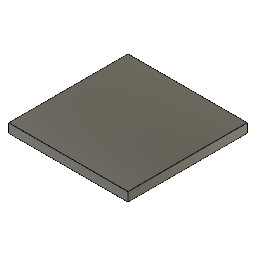
stepper_nema17 v0 (Autodesk Fusion 360 design; units mm, degrees)
Autodesk Fusion 360 part; units mm, degrees
sketch "Sketch1" plane through (0, 0, 0) normal (0, 0, 1) x (1, 0, 0)
  line L0 (21, -21) -> (-21, -21)
  line L1 (-21, -21) -> (-21, 21)
  line L2 (-21, 21) -> (21, 21)
  line L3 (21, 21) -> (21, -21)
  line L4 (21, -21) -> (-21, 21) construction
  line L5 (-21, -21) -> (21, 21) construction
  circle A0 centre (16, -16) radius 1.5
  line L6 (0, 0) -> (21, 0)
  line L7 (0, 0) -> (0, -21)
  line L8 (0, 0) -> (0, 21)
  line L9 (0, 0) -> (-21, 0)
  circle A1 centre (16, 16) radius 1.5
  circle A2 centre (-16, -16) radius 1.5
  circle A3 centre (-16, 16) radius 1.5
  dimension "d1" = 42
  dimension "d2" = 42
  dimension "d3" = 3
  dimension "d4" = 5
  dimension "d5" = 5
  constraint horizontal L0
  constraint perpendicular L0 L1
  constraint parallel L0 L2
  constraint parallel L1 L3
  constraint coincident L4 L6.start
  constraint coincident L5 L6.start
  constraint coincident L6.start L7.start
  constraint midpoint L3 L6.end
  constraint midpoint L0 L7.end
  constraint midpoint L2 L8.end
  constraint midpoint L1 L9.end
  constraint symmetric A0 L6 A1
  constraint symmetric A0 L7 A2
  constraint symmetric L8 A1 A3
  measures "d1" distance of L1.end L2.end
  measures "d2" distance of L0.end L1.end
  measures "d3" diameter of A0
  measures "d4" distance of L0 A0.centre
  measures "d5" distance of L3 A0.centre
extrude "Extrude1" add sketch "Sketch1" against normal blind 40 makes body 1
sketch "Sketch2" plane through (0, 0, 0) normal (0, 0, 1) x (-1, 0, 0)
  circle A0 centre (16, -16) radius 1.5
  circle A1 centre (-16, -16) radius 1.5
  circle A2 centre (-16, 16) radius 1.5
  circle A3 centre (16, 16) radius 1.5
  line L0 (-21, -21) -> (21, -21)
  line L1 (21, -21) -> (21, 21)
  line L2 (21, 21) -> (-21, 21)
  line L3 (-21, 21) -> (-21, -21)
  circle A4 centre (0, 0) radius 11
  dimension "d8" = 22
  constraint coincident A4.centre origin
  measures "d8" diameter of A4
extrude "Extrude2" add sketch "Sketch2" along normal blind 3 contours A4 bodies 1
sketch "Sketch3" plane through (0, 0, 3) normal (0, 0, 1) x (-1, 0, 0)
  circle A0 centre (0, 0) radius 11
  circle A1 centre (0, 0) radius 2.5
  circle A2 centre (0, 0) radius 2
  line L0 (0, -2) -> (1.5, -2)
  line L1 (-1.5, -2) -> (0, -2)
  line L2 (0, 0) -> (0, -2.5)
  dimension "d11" = 5
  dimension "d12" = 4
  constraint coincident A0.centre A1.centre
  constraint concentric A1 A2
  constraint coincident A2 L0.start
  constraint coincident A1 L0.end
  constraint tangent A2 L0
  constraint horizontal L0
  constraint coincident A1 L1.start
  constraint tangent A2 L1
  constraint coincident A1 L2.end
  constraint perpendicular L1 L2
  measures "d11" diameter of A1
  measures "d12" diameter of A2
extrude "Extrude3" add sketch "Sketch3" along normal blind 25 contours A2 | A1 L0 L1 bodies 1
sketch "Sketch4" plane through (0, 0, 0) normal (0, 1, 0) x (1, 0, 0)
sketch "Sketch5" plane through (0, 0, 0) normal (0, 0, 1) x (1, 0, 0)
sketch "Sketch1 (2)" plane through (0, 0, 0) normal (0, 0, 1) x (1, 0, 0) in component "Component"
  line L0 (21.25, 21.25) -> (-21.25, 21.25)
  line L1 (-21.25, 21.25) -> (-21.25, -21.25)
  line L2 (-21.25, -21.25) -> (21.25, -21.25)
  line L3 (21.25, -21.25) -> (21.25, 21.25)
  line L4 (21.25, 21.25) -> (-21.25, -21.25) construction
  line L5 (-21.25, 21.25) -> (21.25, -21.25) construction
  line L6 (22.5, 22.5) -> (-22.5, 22.5)
  line L7 (-22.5, 22.5) -> (-22.5, -22.5)
  line L8 (-22.5, -22.5) -> (22.5, -22.5)
  line L9 (22.5, -22.5) -> (22.5, 22.5)
  line L10 (22.5, 22.5) -> (-22.5, -22.5) construction
  line L11 (-22.5, 22.5) -> (22.5, -22.5) construction
  line L12 (0, 0) -> (0, -21.25)
  line L13 (0, 0) -> (-21.25, 0)
  line L14 (0, 0) -> (0, 21.25)
  line L15 (0, 0) -> (21.25, 0)
  circle A0 centre (17.5, -17.5) radius 1.5
  circle A1 centre (-17.5, -17.5) radius 1.5
  circle A2 centre (17.5, 17.5) radius 1.5
  circle A3 centre (-17.5, 17.5) radius 1.5
  dimension "d15" = 42.5
  dimension "d16" = 42.5
  dimension "d17" = 45
  dimension "d18" = 45
  dimension "d21" = 3
  dimension "d22" = 3.75
  constraint horizontal L0
  constraint perpendicular L0 L1
  constraint parallel L0 L2
  constraint parallel L1 L3
  constraint coincident L4 L12.start
  constraint coincident L5 L12.start
  constraint coincident L12.start L13.start
  constraint horizontal L6
  constraint perpendicular L6 L7
  constraint parallel L6 L8
  constraint parallel L7 L9
  constraint coincident L10 L12.start
  constraint coincident L11 L12.start
  constraint midpoint L2 L12.end
  constraint midpoint L1 L13.end
  constraint midpoint L0 L14.end
  constraint midpoint L3 L15.end
  constraint coincident L5 A0.centre
  constraint symmetric L12 A0 A1
  constraint symmetric L15 A0 A2
  constraint symmetric L14 A2 A3
  measures "d15" distance of L1.end L2.end
  measures "d16" distance of L0.end L1.end
  measures "d17" distance of L7.end L8.end
  measures "d18" distance of L6.end L7.end
  measures "d21" diameter of A0
  measures "d22" distance of L2 A0.centre
extrude "Extrude1'" add sketch "Sketch1 (2)" along normal blind 3.5 separate body contours L0 L3 L14 L15 | L0 L1 L13 L14 | L2 L3 L12 L15 | L1 L2 L12 L13 | L6 L7 L8 L9 | A0 | A1 | A2 | A3 makes body 2 in component "Component"
component "Component" placed x (1, 0, 0) y (0, 1, 0) z (0, 0, 1) at (0, 0, 0)
